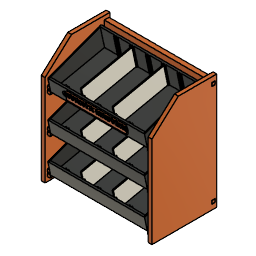
binstack-print-assembly (Autodesk Fusion 360 design; units mm, degrees)
part number: 2026-08-18-19-37-01-070
part number: 2026-08-18-19-37-02-424
part number: 2026-08-18-19-37-02-712
part number: 2026-08-18-19-37-03-090
part number: 2026-08-18-19-37-04-075
part number: 2026-08-18-19-37-04-467
part number: 2026-08-18-19-37-04-536
Autodesk Fusion 360 part; units mm, degrees
sketch "Sketch1" plane through (0, 0, 0) normal (1, 0, 0) x (0, 0, -1) in component "Боковина левая"
  line L0 (0, 15) -> (0, 150)
  line L1 (0, 150) -> (-240, 150)
  line L2 (-240, 150) -> (-240, 70)
  line L3 (-240, 70) -> (-190, 15)
  line L4 (-190, 15) -> (0, 15)
extrude "Extrude1" add sketch "Sketch1" along normal blind 8 makes body 1 in component "Боковина левая"
sketch "Sketch2" plane through (0, 0, 0) normal (1, 0, 0) x (0, 0, -1) in component "Боковина левая"
  line L0 (-9, 20) -> (-35.5696, 145)
  line L1 (-35.5696, 145) -> (-41.5696, 145)
  line L2 (-41.5696, 145) -> (-15, 20)
  line L3 (-15, 20) -> (-9, 20)
extrude "Extrude2" add sketch "Sketch2" along normal blind 6 from surface at 8 separate body makes body 2 in component "Боковина левая"
sketch "Sketch3" plane through (0, 0, 0) normal (1, 0, 0) x (0, 0, -1) in component "Боковина левая"
  line L0 (-18.2, 20) -> (-44.7696, 145)
  line L1 (-44.7696, 145) -> (-49.7696, 145)
  line L2 (-49.7696, 145) -> (-23.2, 20)
  line L3 (-23.2, 20) -> (-18.2, 20)
extrude "Extrude3" add sketch "Sketch3" along normal blind 6 from surface at 8 separate body makes body 3 in component "Боковина левая"
sketch "Sketch4" plane through (0, 0, 0) normal (1, 0, 0) x (0, 0, -1) in component "Боковина левая"
  line L0 (-16.2753, 26) -> (-16.9753, 28)
  line L1 (-16.9753, 28) -> (-18.0381, 31)
  line L2 (-18.0381, 31) -> (-17.7632, 33)
  line L3 (-17.7632, 33) -> (-16.2753, 26)
extrude "Extrude4" add sketch "Sketch4" along normal blind 6 from surface at 8 separate body makes body 4 in component "Боковина левая"
sketch "Sketch5" plane through (0, 0, 0) normal (1, 0, 0) x (0, 0, -1) in component "Боковина левая"
  line L0 (-84, 20) -> (-110.5696, 145)
  line L1 (-110.5696, 145) -> (-116.5696, 145)
  line L2 (-116.5696, 145) -> (-90, 20)
  line L3 (-90, 20) -> (-84, 20)
extrude "Extrude5" add sketch "Sketch5" along normal blind 6 from surface at 8 separate body makes body 5 in component "Боковина левая"
sketch "Sketch6" plane through (0, 0, 0) normal (1, 0, 0) x (0, 0, -1) in component "Боковина левая"
  line L0 (-93.2, 20) -> (-119.7696, 145)
  line L1 (-119.7696, 145) -> (-124.7696, 145)
  line L2 (-124.7696, 145) -> (-98.2, 20)
  line L3 (-98.2, 20) -> (-93.2, 20)
extrude "Extrude6" add sketch "Sketch6" along normal blind 6 from surface at 8 separate body makes body 6 in component "Боковина левая"
sketch "Sketch7" plane through (0, 0, 0) normal (1, 0, 0) x (0, 0, -1) in component "Боковина левая"
  line L0 (-91.2753, 26) -> (-91.9753, 28)
  line L1 (-91.9753, 28) -> (-93.0381, 31)
  line L2 (-93.0381, 31) -> (-92.7632, 33)
  line L3 (-92.7632, 33) -> (-91.2753, 26)
extrude "Extrude7" add sketch "Sketch7" along normal blind 6 from surface at 8 separate body makes body 7 in component "Боковина левая"
sketch "Sketch8" plane through (0, 0, 0) normal (1, 0, 0) x (0, 0, -1) in component "Боковина левая"
  line L0 (-159, 20) -> (-185.5696, 145)
  line L1 (-185.5696, 145) -> (-191.5696, 145)
  line L2 (-191.5696, 145) -> (-165, 20)
  line L3 (-165, 20) -> (-159, 20)
extrude "Extrude8" add sketch "Sketch8" along normal blind 6 from surface at 8 separate body makes body 8 in component "Боковина левая"
sketch "Sketch9" plane through (0, 0, 0) normal (1, 0, 0) x (0, 0, -1) in component "Боковина левая"
  line L0 (-168.2, 20) -> (-194.7696, 145)
  line L1 (-194.7696, 145) -> (-199.7696, 145)
  line L2 (-199.7696, 145) -> (-173.2, 20)
  line L3 (-173.2, 20) -> (-168.2, 20)
extrude "Extrude9" add sketch "Sketch9" along normal blind 6 from surface at 8 separate body makes body 9 in component "Боковина левая"
sketch "Sketch10" plane through (0, 0, 0) normal (1, 0, 0) x (0, 0, -1) in component "Боковина левая"
  line L0 (-166.2753, 26) -> (-166.9753, 28)
  line L1 (-166.9753, 28) -> (-168.0381, 31)
  line L2 (-168.0381, 31) -> (-167.7632, 33)
  line L3 (-167.7632, 33) -> (-166.2753, 26)
extrude "Extrude10" add sketch "Sketch10" along normal blind 6 from surface at 8 separate body makes body 10 in component "Боковина левая"
combine "Combine1" operation add target body 1 tool bodies 2 3 4 5 6 7 8 9 10 in component "Боковина левая"
sketch "Sketch11" plane through (0, 0, 0) normal (1, 0, 0) x (0, 0, -1) in component "Боковина левая"
  line L0 (-10.5, 139.5) -> (-10.5, 146.5)
  line L1 (-10.5, 146.5) -> (-17.5, 146.5)
  line L2 (-17.5, 146.5) -> (-17.5, 139.5)
  line L3 (-17.5, 139.5) -> (-10.5, 139.5)
extrude "Extrude11" cut sketch "Sketch11" along normal blind 30 from surface at -2 bodies 1 in component "Боковина левая"
sketch "Sketch12" plane through (0, 0, 0) normal (1, 0, 0) x (0, 0, -1) in component "Боковина левая"
  line L0 (-222.5, 139.5) -> (-222.5, 146.5)
  line L1 (-222.5, 146.5) -> (-229.5, 146.5)
  line L2 (-229.5, 146.5) -> (-229.5, 139.5)
  line L3 (-229.5, 139.5) -> (-222.5, 139.5)
extrude "Extrude12" cut sketch "Sketch12" along normal blind 30 from surface at -2 bodies 1 in component "Боковина левая"
sketch "Sketch1 (2)" plane through (0, 0, 0) normal (1, 0, 0) x (0, 0, -1) in component "Боковина правая"
  line L0 (0, 15) -> (0, 150)
  line L1 (0, 150) -> (-240, 150)
  line L2 (-240, 150) -> (-240, 70)
  line L3 (-240, 70) -> (-190, 15)
  line L4 (-190, 15) -> (0, 15)
extrude "Extrude1'" add sketch "Sketch1 (2)" along normal blind 8 from surface at 6 separate body makes body 11 in component "Боковина правая"
sketch "Sketch2 (2)" plane through (0, 0, 0) normal (1, 0, 0) x (0, 0, -1) in component "Боковина правая"
  line L0 (-9, 20) -> (-35.5696, 145)
  line L1 (-35.5696, 145) -> (-41.5696, 145)
  line L2 (-41.5696, 145) -> (-15, 20)
  line L3 (-15, 20) -> (-9, 20)
extrude "Extrude2'" add sketch "Sketch2 (2)" along normal blind 6 separate body makes body 12 in component "Боковина правая"
sketch "Sketch3 (2)" plane through (0, 0, 0) normal (1, 0, 0) x (0, 0, -1) in component "Боковина правая"
  line L0 (-18.2, 20) -> (-44.7696, 145)
  line L1 (-44.7696, 145) -> (-49.7696, 145)
  line L2 (-49.7696, 145) -> (-23.2, 20)
  line L3 (-23.2, 20) -> (-18.2, 20)
extrude "Extrude3'" add sketch "Sketch3 (2)" along normal blind 6 separate body makes body 13 in component "Боковина правая"
sketch "Sketch4 (2)" plane through (0, 0, 0) normal (1, 0, 0) x (0, 0, -1) in component "Боковина правая"
  line L0 (-16.2753, 26) -> (-16.9753, 28)
  line L1 (-16.9753, 28) -> (-18.0381, 31)
  line L2 (-18.0381, 31) -> (-17.7632, 33)
  line L3 (-17.7632, 33) -> (-16.2753, 26)
extrude "Extrude4'" add sketch "Sketch4 (2)" along normal blind 6 separate body makes body 14 in component "Боковина правая"
sketch "Sketch5 (2)" plane through (0, 0, 0) normal (1, 0, 0) x (0, 0, -1) in component "Боковина правая"
  line L0 (-84, 20) -> (-110.5696, 145)
  line L1 (-110.5696, 145) -> (-116.5696, 145)
  line L2 (-116.5696, 145) -> (-90, 20)
  line L3 (-90, 20) -> (-84, 20)
extrude "Extrude5'" add sketch "Sketch5 (2)" along normal blind 6 separate body makes body 15 in component "Боковина правая"
sketch "Sketch6 (2)" plane through (0, 0, 0) normal (1, 0, 0) x (0, 0, -1) in component "Боковина правая"
  line L0 (-93.2, 20) -> (-119.7696, 145)
  line L1 (-119.7696, 145) -> (-124.7696, 145)
  line L2 (-124.7696, 145) -> (-98.2, 20)
  line L3 (-98.2, 20) -> (-93.2, 20)
extrude "Extrude6'" add sketch "Sketch6 (2)" along normal blind 6 separate body makes body 16 in component "Боковина правая"
sketch "Sketch7 (2)" plane through (0, 0, 0) normal (1, 0, 0) x (0, 0, -1) in component "Боковина правая"
  line L0 (-91.2753, 26) -> (-91.9753, 28)
  line L1 (-91.9753, 28) -> (-93.0381, 31)
  line L2 (-93.0381, 31) -> (-92.7632, 33)
  line L3 (-92.7632, 33) -> (-91.2753, 26)
extrude "Extrude7'" add sketch "Sketch7 (2)" along normal blind 6 separate body makes body 17 in component "Боковина правая"
sketch "Sketch8 (2)" plane through (0, 0, 0) normal (1, 0, 0) x (0, 0, -1) in component "Боковина правая"
  line L0 (-159, 20) -> (-185.5696, 145)
  line L1 (-185.5696, 145) -> (-191.5696, 145)
  line L2 (-191.5696, 145) -> (-165, 20)
  line L3 (-165, 20) -> (-159, 20)
extrude "Extrude8'" add sketch "Sketch8 (2)" along normal blind 6 separate body makes body 18 in component "Боковина правая"
sketch "Sketch9 (2)" plane through (0, 0, 0) normal (1, 0, 0) x (0, 0, -1) in component "Боковина правая"
  line L0 (-168.2, 20) -> (-194.7696, 145)
  line L1 (-194.7696, 145) -> (-199.7696, 145)
  line L2 (-199.7696, 145) -> (-173.2, 20)
  line L3 (-173.2, 20) -> (-168.2, 20)
extrude "Extrude9'" add sketch "Sketch9 (2)" along normal blind 6 separate body makes body 19 in component "Боковина правая"
sketch "Sketch10 (2)" plane through (0, 0, 0) normal (1, 0, 0) x (0, 0, -1) in component "Боковина правая"
  line L0 (-166.2753, 26) -> (-166.9753, 28)
  line L1 (-166.9753, 28) -> (-168.0381, 31)
  line L2 (-168.0381, 31) -> (-167.7632, 33)
  line L3 (-167.7632, 33) -> (-166.2753, 26)
extrude "Extrude10'" add sketch "Sketch10 (2)" along normal blind 6 separate body makes body 20 in component "Боковина правая"
combine "Combine1'" operation add target body 11 tool bodies 12 13 14 15 16 17 18 19 20 in component "Боковина правая"
sketch "Sketch11 (2)" plane through (0, 0, 0) normal (1, 0, 0) x (0, 0, -1) in component "Боковина правая"
  line L0 (-10.5, 139.5) -> (-10.5, 146.5)
  line L1 (-10.5, 146.5) -> (-17.5, 146.5)
  line L2 (-17.5, 146.5) -> (-17.5, 139.5)
  line L3 (-17.5, 139.5) -> (-10.5, 139.5)
extrude "Extrude11'" cut sketch "Sketch11 (2)" along normal blind 30 from surface at -2 bodies 11 in component "Боковина правая"
sketch "Sketch12 (2)" plane through (0, 0, 0) normal (1, 0, 0) x (0, 0, -1) in component "Боковина правая"
  line L0 (-222.5, 139.5) -> (-222.5, 146.5)
  line L1 (-222.5, 146.5) -> (-229.5, 146.5)
  line L2 (-229.5, 146.5) -> (-229.5, 139.5)
  line L3 (-229.5, 139.5) -> (-222.5, 139.5)
extrude "Extrude12'" cut sketch "Sketch12 (2)" along normal blind 30 from surface at -2 bodies 11 in component "Боковина правая"
sketch "Sketch1 (3)" plane through (0, 0, 0) normal (0, 0, 1) x (1, 0, 0) in component "Лоток"
  line L0 (-6, 0) -> (207, 0)
  line L1 (207, 0) -> (207, 117)
  line L2 (207, 117) -> (-6, 117)
  line L3 (-6, 117) -> (-6, 0)
extrude "Extrude1''" add sketch "Sketch1 (3)" along normal blind 2.4 separate body makes body 21 in component "Лоток"
sketch "Sketch2 (3)" plane through (0, 0, 0) normal (0, 0, 1) x (1, 0, 0) in component "Лоток"
  line L0 (0, 0) -> (201, 0)
  line L1 (201, 0) -> (201, 4)
  line L2 (201, 4) -> (0, 4)
  line L3 (0, 4) -> (0, 0)
extrude "Extrude2''" add sketch "Sketch2 (3)" along normal blind 28 separate body makes body 22 in component "Лоток"
sketch "Sketch3 (3)" plane through (0, 0, 0) normal (0, 0, 1) x (1, 0, 0) in component "Лоток"
  line L0 (0, 113) -> (201, 113)
  line L1 (201, 113) -> (201, 117)
  line L2 (201, 117) -> (0, 117)
  line L3 (0, 117) -> (0, 113)
extrude "Extrude3''" add sketch "Sketch3 (3)" along normal blind 45 separate body makes body 23 in component "Лоток"
sketch "Sketch4 (3)" plane through (0, 0, 0) normal (1, 0, 0) x (0, 0, -1) in component "Лоток"
  line L0 (0, 0) -> (0, 117)
  line L1 (0, 117) -> (-45, 117)
  line L2 (-45, 117) -> (-28, 0)
  line L3 (-28, 0) -> (0, 0)
extrude "Extrude4''" add sketch "Sketch4 (3)" along normal blind 2 separate body makes body 24 in component "Лоток"
sketch "Sketch5 (3)" plane through (0, 0, 0) normal (1, 0, 0) x (0, 0, -1) in component "Лоток"
  line L0 (0, 0) -> (0, 117)
  line L1 (0, 117) -> (-45, 117)
  line L2 (-45, 117) -> (-28, 0)
  line L3 (-28, 0) -> (0, 0)
extrude "Extrude5''" add sketch "Sketch5 (3)" along normal blind 2 from surface at 199 separate body makes body 25 in component "Лоток"
sketch "Sketch6 (3)" plane through (0, 0, 0) normal (0, 0, 1) x (1, 0, 0) in component "Лоток"
  line L0 (31.4, 4) -> (33.4, 4)
  line L1 (33.4, 4) -> (33.4, 6)
  line L2 (33.4, 6) -> (31.4, 6)
  line L3 (31.4, 6) -> (31.4, 4)
extrude "Extrude6''" add sketch "Sketch6 (3)" along normal blind 25.6 from surface at 2.4 separate body makes body 26 in component "Лоток"
sketch "Sketch7 (3)" plane through (0, 0, 0) normal (0, 0, 1) x (1, 0, 0) in component "Лоток"
  line L0 (31.4, 111) -> (33.4, 111)
  line L1 (33.4, 111) -> (33.4, 113)
  line L2 (33.4, 113) -> (31.4, 113)
  line L3 (31.4, 113) -> (31.4, 111)
extrude "Extrude7''" add sketch "Sketch7 (3)" along normal blind 42.6 from surface at 2.4 separate body makes body 27 in component "Лоток"
sketch "Sketch8 (3)" plane through (0, 0, 0) normal (0, 0, 1) x (1, 0, 0) in component "Лоток"
  line L0 (36.6, 4) -> (38.6, 4)
  line L1 (38.6, 4) -> (38.6, 6)
  line L2 (38.6, 6) -> (36.6, 6)
  line L3 (36.6, 6) -> (36.6, 4)
extrude "Extrude8''" add sketch "Sketch8 (3)" along normal blind 25.6 from surface at 2.4 separate body makes body 28 in component "Лоток"
sketch "Sketch9 (3)" plane through (0, 0, 0) normal (0, 0, 1) x (1, 0, 0) in component "Лоток"
  line L0 (36.6, 111) -> (38.6, 111)
  line L1 (38.6, 111) -> (38.6, 113)
  line L2 (38.6, 113) -> (36.6, 113)
  line L3 (36.6, 113) -> (36.6, 111)
extrude "Extrude9''" add sketch "Sketch9 (3)" along normal blind 42.6 from surface at 2.4 separate body makes body 29 in component "Лоток"
sketch "Sketch10 (3)" plane through (0, 0, 0) normal (0, 0, 1) x (1, 0, 0) in component "Лоток"
  line L0 (64.4, 4) -> (66.4, 4)
  line L1 (66.4, 4) -> (66.4, 6)
  line L2 (66.4, 6) -> (64.4, 6)
  line L3 (64.4, 6) -> (64.4, 4)
extrude "Extrude10''" add sketch "Sketch10 (3)" along normal blind 25.6 from surface at 2.4 separate body makes body 30 in component "Лоток"
sketch "Sketch11 (3)" plane through (0, 0, 0) normal (0, 0, 1) x (1, 0, 0) in component "Лоток"
  line L0 (64.4, 111) -> (66.4, 111)
  line L1 (66.4, 111) -> (66.4, 113)
  line L2 (66.4, 113) -> (64.4, 113)
  line L3 (64.4, 113) -> (64.4, 111)
extrude "Extrude11''" add sketch "Sketch11 (3)" along normal blind 42.6 from surface at 2.4 separate body makes body 31 in component "Лоток"
sketch "Sketch12 (3)" plane through (0, 0, 0) normal (0, 0, 1) x (1, 0, 0) in component "Лоток"
  line L0 (69.6, 4) -> (71.6, 4)
  line L1 (71.6, 4) -> (71.6, 6)
  line L2 (71.6, 6) -> (69.6, 6)
  line L3 (69.6, 6) -> (69.6, 4)
extrude "Extrude12''" add sketch "Sketch12 (3)" along normal blind 25.6 from surface at 2.4 separate body makes body 32 in component "Лоток"
sketch "Sketch13" plane through (0, 0, 0) normal (0, 0, 1) x (1, 0, 0) in component "Лоток"
  line L0 (69.6, 111) -> (71.6, 111)
  line L1 (71.6, 111) -> (71.6, 113)
  line L2 (71.6, 113) -> (69.6, 113)
  line L3 (69.6, 113) -> (69.6, 111)
extrude "Extrude13" add sketch "Sketch13" along normal blind 42.6 from surface at 2.4 separate body makes body 33 in component "Лоток"
sketch "Sketch14" plane through (0, 0, 0) normal (0, 0, 1) x (1, 0, 0) in component "Лоток"
  line L0 (97.4, 4) -> (99.4, 4)
  line L1 (99.4, 4) -> (99.4, 6)
  line L2 (99.4, 6) -> (97.4, 6)
  line L3 (97.4, 6) -> (97.4, 4)
extrude "Extrude14" add sketch "Sketch14" along normal blind 25.6 from surface at 2.4 separate body makes body 34 in component "Лоток"
sketch "Sketch15" plane through (0, 0, 0) normal (0, 0, 1) x (1, 0, 0) in component "Лоток"
  line L0 (97.4, 111) -> (99.4, 111)
  line L1 (99.4, 111) -> (99.4, 113)
  line L2 (99.4, 113) -> (97.4, 113)
  line L3 (97.4, 113) -> (97.4, 111)
extrude "Extrude15" add sketch "Sketch15" along normal blind 42.6 from surface at 2.4 separate body makes body 35 in component "Лоток"
sketch "Sketch16" plane through (0, 0, 0) normal (0, 0, 1) x (1, 0, 0) in component "Лоток"
  line L0 (102.6, 4) -> (104.6, 4)
  line L1 (104.6, 4) -> (104.6, 6)
  line L2 (104.6, 6) -> (102.6, 6)
  line L3 (102.6, 6) -> (102.6, 4)
extrude "Extrude16" add sketch "Sketch16" along normal blind 25.6 from surface at 2.4 separate body makes body 36 in component "Лоток"
sketch "Sketch17" plane through (0, 0, 0) normal (0, 0, 1) x (1, 0, 0) in component "Лоток"
  line L0 (102.6, 111) -> (104.6, 111)
  line L1 (104.6, 111) -> (104.6, 113)
  line L2 (104.6, 113) -> (102.6, 113)
  line L3 (102.6, 113) -> (102.6, 111)
extrude "Extrude17" add sketch "Sketch17" along normal blind 42.6 from surface at 2.4 separate body makes body 37 in component "Лоток"
sketch "Sketch18" plane through (0, 0, 0) normal (0, 0, 1) x (1, 0, 0) in component "Лоток"
  line L0 (130.4, 4) -> (132.4, 4)
  line L1 (132.4, 4) -> (132.4, 6)
  line L2 (132.4, 6) -> (130.4, 6)
  line L3 (130.4, 6) -> (130.4, 4)
extrude "Extrude18" add sketch "Sketch18" along normal blind 25.6 from surface at 2.4 separate body makes body 38 in component "Лоток"
sketch "Sketch19" plane through (0, 0, 0) normal (0, 0, 1) x (1, 0, 0) in component "Лоток"
  line L0 (130.4, 111) -> (132.4, 111)
  line L1 (132.4, 111) -> (132.4, 113)
  line L2 (132.4, 113) -> (130.4, 113)
  line L3 (130.4, 113) -> (130.4, 111)
extrude "Extrude19" add sketch "Sketch19" along normal blind 42.6 from surface at 2.4 separate body makes body 39 in component "Лоток"
sketch "Sketch20" plane through (0, 0, 0) normal (0, 0, 1) x (1, 0, 0) in component "Лоток"
  line L0 (135.6, 4) -> (137.6, 4)
  line L1 (137.6, 4) -> (137.6, 6)
  line L2 (137.6, 6) -> (135.6, 6)
  line L3 (135.6, 6) -> (135.6, 4)
extrude "Extrude20" add sketch "Sketch20" along normal blind 25.6 from surface at 2.4 separate body makes body 40 in component "Лоток"
sketch "Sketch21" plane through (0, 0, 0) normal (0, 0, 1) x (1, 0, 0) in component "Лоток"
  line L0 (135.6, 111) -> (137.6, 111)
  line L1 (137.6, 111) -> (137.6, 113)
  line L2 (137.6, 113) -> (135.6, 113)
  line L3 (135.6, 113) -> (135.6, 111)
extrude "Extrude21" add sketch "Sketch21" along normal blind 42.6 from surface at 2.4 separate body makes body 41 in component "Лоток"
sketch "Sketch22" plane through (0, 0, 0) normal (0, 0, 1) x (1, 0, 0) in component "Лоток"
  line L0 (163.4, 4) -> (165.4, 4)
  line L1 (165.4, 4) -> (165.4, 6)
  line L2 (165.4, 6) -> (163.4, 6)
  line L3 (163.4, 6) -> (163.4, 4)
extrude "Extrude22" add sketch "Sketch22" along normal blind 25.6 from surface at 2.4 separate body makes body 42 in component "Лоток"
sketch "Sketch23" plane through (0, 0, 0) normal (0, 0, 1) x (1, 0, 0) in component "Лоток"
  line L0 (163.4, 111) -> (165.4, 111)
  line L1 (165.4, 111) -> (165.4, 113)
  line L2 (165.4, 113) -> (163.4, 113)
  line L3 (163.4, 113) -> (163.4, 111)
extrude "Extrude23" add sketch "Sketch23" along normal blind 42.6 from surface at 2.4 separate body makes body 43 in component "Лоток"
sketch "Sketch24" plane through (0, 0, 0) normal (0, 0, 1) x (1, 0, 0) in component "Лоток"
  line L0 (168.6, 4) -> (170.6, 4)
  line L1 (170.6, 4) -> (170.6, 6)
  line L2 (170.6, 6) -> (168.6, 6)
  line L3 (168.6, 6) -> (168.6, 4)
extrude "Extrude24" add sketch "Sketch24" along normal blind 25.6 from surface at 2.4 separate body makes body 44 in component "Лоток"
sketch "Sketch25" plane through (0, 0, 0) normal (0, 0, 1) x (1, 0, 0) in component "Лоток"
  line L0 (168.6, 111) -> (170.6, 111)
  line L1 (170.6, 111) -> (170.6, 113)
  line L2 (170.6, 113) -> (168.6, 113)
  line L3 (168.6, 113) -> (168.6, 111)
extrude "Extrude25" add sketch "Sketch25" along normal blind 42.6 from surface at 2.4 separate body makes body 45 in component "Лоток"
combine "Combine1''" operation add target body 21 tool bodies 22 23 24 25 26 27 28 29 30 31 32 33 34 35 36 37 38 39 40 41 42 43 44 45 in component "Лоток"
sketch "Sketch1 (4)" plane through (0, 0, 0) normal (0, 0, 1) x (1, 0, 0) in component "Планка логотипа"
  line L0 (0, 0) -> (125, 0)
  line L1 (125, 0) -> (125, 3)
  line L2 (125, 3) -> (0, 3)
  line L3 (0, 3) -> (0, 0)
extrude "Extrude1'''" add sketch "Sketch1 (4)" along normal blind 17 separate body makes body 46 in component "Планка логотипа"
sketch "Sketch2 (4)" plane through (0, 0, 0) normal (0, -1, 0) x (1, 0, 0) in component "Планка логотипа"
  line L0 (0, 0) -> (125, 0)
  line L1 (125, 0) -> (125, 17)
  line L2 (125, 17) -> (0, 17)
  line L3 (0, 17) -> (0, 0)
  line L4 (8, 8.5) -> (117, 8.5)
  dimension "d151" = 9
  text T0 "GIVANTA MASTERS" font "Arial Black" height 9 align centre spacing 1 along the path L4 letters at x, y, angle (-5.6753, 22.3377, 0) (4.7981, 22.3377, 0) (9.691, 22.3377, 0) (19.4829, 22.3377, 0) (29.2995, 22.3377, 0) (39.7729, 22.3377, 0) (48.8527, 22.3377, 0) (58.6692, 22.3377, 0) (62.8622, 22.3377, 0) (74.7292, 22.3377, 0) (84.5457, 22.3377, 0) (93.6255, 22.3377, 0) (102.7053, 22.3377, 0) (111.7851, 22.3377, 0) (121.5955, 22.3377, 0)
extrude "Extrude2'''" add sketch "Sketch2 (4)" along normal blind 0.8 separate body text T0 makes body 47 at (104.5491, 0, 12.7708) makes body 48 at (64.5116, 0, 13.7879) makes body 49 at (26.854, 0, 12.6439) makes body 50 at (3.2551, 0, 11.7292) makes body 51 at (37.972, 0, 12.8404) makes body 52 at (82.1003, 0, 12.6439) makes body 53 at (113.6739, 0, 12.7176) makes body 54 at (97.6774, 0, 13.0184) makes body 55 at (56.2237, 0, 12.6439) makes body 56 at (12.5007, 0, 12.3411) makes body 57 at (6.7585, 0, 14.5) makes body 58 at (43.8247, 0, 13.0184) makes body 59 at (90.7117, 0, 13.219) makes body 60 at (127.7615, 0, 13.219) in component "Планка логотипа"
sketch "Sketch1 (5)" plane through (0, 0, 0) normal (0, 0, 1) x (1, 0, 0) in component "Перегородка"
  line L0 (0, 0) -> (2.4, 0)
  line L1 (2.4, 0) -> (2.4, 109)
  line L2 (2.4, 109) -> (0, 109)
  line L3 (0, 109) -> (0, 0)
extrude "Extrude1''''" add sketch "Sketch1 (5)" along normal blind 40 separate body makes body 61 in component "Перегородка"
sketch "Sketch1 (6)" plane through (0, 0, 0) normal (0, 0, 1) x (1, 0, 0) in component "Штанга"
  line L0 (0, 0) -> (214, 0)
  line L1 (214, 0) -> (214, 10)
  line L2 (214, 10) -> (0, 10)
  line L3 (0, 10) -> (0, 0)
extrude "Extrude1'''''" add sketch "Sketch1 (6)" along normal blind 12 separate body makes body 62 in component "Штанга"
sketch "Sketch2 (5)" plane through (0, 0, 0) normal (0, 0, 1) x (1, 0, 0) in component "Штанга"
  line L0 (-8, 2) -> (0, 2)
  line L1 (0, 2) -> (0, 8)
  line L2 (0, 8) -> (-8, 8)
  line L3 (-8, 8) -> (-8, 2)
extrude "Extrude2''''" add sketch "Sketch2 (5)" along normal blind 6 from surface at 3 separate body makes body 63 in component "Штанга"
sketch "Sketch3 (4)" plane through (0, 0, 0) normal (0, 0, 1) x (1, 0, 0) in component "Штанга"
  line L0 (214, 2) -> (222, 2)
  line L1 (222, 2) -> (222, 8)
  line L2 (222, 8) -> (214, 8)
  line L3 (214, 8) -> (214, 2)
extrude "Extrude3'''" add sketch "Sketch3 (4)" along normal blind 6 from surface at 3 separate body makes body 64 in component "Штанга"
combine "Combine1'''" operation add target body 62 tool bodies 63 64 in component "Штанга"
component "Боковина левая" placed x (1, 0, 0) y (0, 1, 0) z (0, 0, 1) at (0, 0, 0)
component "Боковина правая" placed x (1, 0, 0) y (0, 1, 0) z (0, 0, 1) at (216, 0, 0)
component "Лоток" placed x (1, 0, 0) y (0, 0.978148, 0.207912) z (0, -0.207912, 0.978148) at (14.5, 20, 15)
component "Планка логотипа" placed x (1, 0, 0) y (0, 0.978148, 0.207912) z (0, -0.207912, 0.978148) at (52.5, 15.6102, 171.2233)
component "Перегородка" placed x (1, 0, 0) y (0, 0.978148, 0.207912) z (0, -0.207912, 0.978148) at (81.3, 23.4136, 18.1792)
component "Штанга" placed x (1, 0, 0) y (0, 1, 0) z (0, 0, 1) at (8, 138, 8)
component "Лоток" placed x (1, 0, 0) y (0, 0.978148, 0.207912) z (0, -0.207912, 0.978148) at (14.5, 20, 90)
component "Лоток" placed x (1, 0, 0) y (0, 0.978148, 0.207912) z (0, -0.207912, 0.978148) at (14.5, 20, 165)
component "Перегородка" placed x (1, 0, 0) y (0, 0.978148, 0.207912) z (0, -0.207912, 0.978148) at (147.3, 23.4136, 18.1792)
component "Перегородка" placed x (1, 0, 0) y (0, 0.978148, 0.207912) z (0, -0.207912, 0.978148) at (81.3, 23.4136, 93.1792)
component "Перегородка" placed x (1, 0, 0) y (0, 0.978148, 0.207912) z (0, -0.207912, 0.978148) at (147.3, 23.4136, 93.1792)
component "Перегородка" placed x (1, 0, 0) y (0, 0.978148, 0.207912) z (0, -0.207912, 0.978148) at (81.3, 23.4136, 168.1792)
component "Перегородка" placed x (1, 0, 0) y (0, 0.978148, 0.207912) z (0, -0.207912, 0.978148) at (147.3, 23.4136, 168.1792)
component "Штанга" placed x (1, 0, 0) y (0, 1, 0) z (0, 0, 1) at (8, 138, 220)
equation "d152 = 'GIVANTA MASTERS'"
named bodies: "Тело", "Логотип (2-й цвет)", "Логотип", "Логотип (1)", "Логотип (2)", "Логотип (3)", "Логотип (4)", "Логотип (5)", "Логотип (6)", "Логотип (7)", "Логотип (8)", "Логотип (9)", "Логотип (10)", "Логотип (11)", "Логотип (12)"
